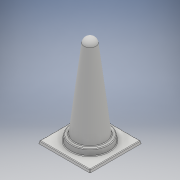
# Autodesk Inventor part: corn
Saved by Autodesk Inventor 2018.2 (Build 222227000, 227)
## iProperties
Created: 2017-12-21
Part Number: corn
Material: 一般
Document SubType Name: Modeling
Designer: ku_sk
Density: 1 g/cm^3
Appearance: 既定
Author: ku_sk
## iProperties of the stored document corn_3D プリント.ipt
Created: 2017-12-21
Part Number: corn_3D プリント
Material: 一般
Document SubType Name: Modeling
Designer: ku_sk
Density: 1 g/cm^3
Appearance: 既定
Author: ku_sk
Autodesk Inventor part; units mm, degrees
ref_plane "YZ Plane" through (0, 0, 0) normal (1, 0, 0) x (0, 1, 0)
ref_plane "XZ Plane" through (0, 0, 0) normal (0, 1, 0) x (-1, 0, 0)
ref_plane "XY Plane" through (0, 0, 0) normal (0, 0, 1) x (1, 0, 0)
sketch "スケッチ1" plane through (0, 0, 0) normal (0, 1, 0) x (-1, 0, 0)
  line L0 (0, -141.7333) -> (0, 850.3995) projected
  line L1 (0, 19) -> (-145, 19)
  line L2 (-145, 19) -> (-140, 62)
  line L3 (-140, 62) -> (0, 62)
  line L4 (-45.528, 659.4592) -> (-115, 62)
  arc A0 (0, 700) -> (-45.528, 659.4592) centre (0, 654.1652) ccw
  point P0 (0, 0)
  dimension "d0" = 145
  dimension "d2" = 43
  dimension "d3" = 19
  dimension "d4" = 115
  dimension "d5" = 700
  dimension "d7" = 5
  constraints: 8 end point, 4 point on line, 2 point on circle, 1 centre point, 1 horizontal, 1 line through centre, 1 parallel, 1 perpendicular, 1 tangent
  measures "d0" distance of L1.start L1.end
  measures "d2" distance between parallel lines of L1 L3
  measures "d3" distance from line of point (0, 0) L1
  measures "d4" distance from line of L0 L4.end
  measures "d5" distance of point (0, 0) A0.start
  measures "d7" horizontal distance of L1.end L2.end
revolve "回転1" add sketch "スケッチ1" angle 360 about axis through (0, 0, -10) along (0, 0, 1)
sketch "スケッチ2" plane through (0, 0, 0) normal (0, 0, 1) x (1, 0, 0)
  line L0 (-195, 195) -> (195, 195)
  line L1 (195, 195) -> (195, -195)
  line L2 (195, -195) -> (-195, -195)
  line L3 (-195, -195) -> (-195, 195)
  line L4 (-195, 195) -> (195, -195) construction
  line L5 (195, 195) -> (-195, -195) construction
  point P0 (0, 0)
  dimension "d9" = 390
  dimension "d10" = 390
  constraints: 12 end point, 2 midpoint, 2 parallel, 1 horizontal, 1 perpendicular
  measures "d9" distance of L0.start L0.end
  measures "d10" distance of L2.end L0.start
extrude "押し出し1" add sketch "スケッチ2" along normal blind 19
chamfer "面取り1" distance 5 distance2 19 1 edges at (195, 0, 19) measured on face at (-2.8103, 178.2516, 19)
chamfer "面取り2" distance 5 distance2 19 1 edges at (-2.5, -195, 19) measured on face at (-178.3333, 0, 19)
chamfer "面取り3" distance 5 distance2 19 1 edges at (-2.4999, 195, 19) measured on face at (-4.477, 178.2516, 19)
chamfer "面取り4" distance 5 distance2 19 1 edges at (-195, 0, 19) measured on face at (-178.3333, 0, 19)
fillet "フィレット1" radius 5 11 edges at (-115, 0, 62) (-140, 0, 62) (-145, 0, 19) (0, -190.0001, 19) (-190.0001, 0, 19) (0, 190.0001, 19) (190.0001, 0, 19) (192.5, 192.5, 9.5) (192.5, -192.5, 9.5) (-192.5001, -192.5, 9.5) (-192.5001, 192.5, 9.5001)
shell "シェル1" thickness 2.5 removed faces 1 at (63.3937, -65, 0)
equation "\"d10\" = d9"
